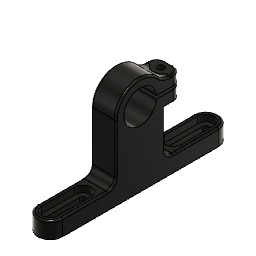
fixation (Autodesk Fusion 360 design; units mm, degrees)
Autodesk Fusion 360 part; units mm, degrees
sketch "Esquisse1" plane through (0, 0, 0) normal (1, 0, 0) x (0, 0, -1)
  circle A0 centre (0, 0) radius 10 construction
  circle A1 centre (0, 0) radius 15 construction
  line L0 (15, -35) -> (15, 0) construction
  line L1 (-15, -35) -> (-15, 0) construction
  line L2 (4, 1) -> (25, 1) construction
  line L3 (4, -1) -> (25, -1) construction
  line L4 (25, -1) -> (25, -7) construction
  line L5 (25, -7) -> (13.2665, -7) construction
  line L6 (25, 1) -> (25, 7) construction
  line L7 (25, 7) -> (13.2665, 7) construction
  line L8 (-15, -35) -> (-55, -35) construction
  line L9 (-55, -35) -> (-55, -45) construction
  line L10 (15, -35) -> (55, -35) construction
  line L11 (55, -35) -> (55, -45) construction
  line L12 (55, -45) -> (-55, -45) construction
  line L13 (55, -45) -> (-55, -45)
  line L14 (-55, -45) -> (-55, -35)
  line L15 (-55, -35) -> (-15, -35)
  line L16 (-15, -35) -> (-15, 0)
  line L17 (13.2665, 7) -> (25, 7)
  line L18 (25, 7) -> (25, 1)
  line L19 (25, 1) -> (9.9499, 1)
  line L20 (9.9499, -1) -> (25, -1)
  line L21 (25, -1) -> (25, -7)
  line L22 (25, -7) -> (15, -7)
  line L23 (15, -7) -> (15, -35)
  line L24 (15, -35) -> (55, -35)
  line L25 (55, -35) -> (55, -45)
  arc A2 (13.2665, 7) -> (-15, 0) centre (0, 0) ccw
  arc A3 (9.9499, 1) -> (9.9499, -1) centre (0, 0) ccw
  dimension "d58" = 20
  dimension "d59" = 30
  dimension "d60" = 10
  dimension "d61" = 10
  dimension "d62" = 45
  dimension "d63" = 10
  dimension "d64" = 10
  constraint coincident A0.centre A1.centre
  constraint coincident A1 L0.end
  constraint tangent A1 L0
  constraint vertical L0
  constraint coincident A1 L1.end
  constraint tangent A1 L1
  constraint parallel L0 L1
  constraint perpendicular L0 L2
  constraint horizontal L3
  constraint perpendicular L3 L4
  constraint coincident A1 L5.end
  constraint perpendicular L0 L5
  constraint perpendicular L2 L6
  constraint coincident A1 L7.end
  constraint perpendicular L6 L7
  constraint perpendicular L1 L8
  constraint perpendicular L8 L9
  constraint perpendicular L0 L10
  constraint perpendicular L10 L11
  constraint parallel L12 L13
  constraint coincident A0 L19.end
  constraint coincident L2 L19.end
  constraint coincident A0 L20.start
  constraint coincident L3 L20.start
  constraint coincident L5 L22.end
  constraint coincident L0 L22.end
  constraint parallel L11 L25
  measures "d58" diameter of A0
  measures "d59" diameter of A1
  measures "d60" distance of L0 L2.end
  measures "d61" distance of L0 L3.end
  measures "d62" distance of A0.centre L12
  measures "d63" distance of L10 L12
  measures "d64" distance of L8 L12
extrude "Extrusion8" add sketch "Esquisse1" along normal blind 15
fillet "Congé9" radius 7.5 4 edges at (15, -40, -55) (0, -40, -55) (15, -40, 55) (0, -40, 55)
fillet "Congé10" radius 5 2 edges at (7.5, -35, -15) (7.5, -35, 15)
sketch "Esquisse8" plane through (0, -35, 0) normal (0, 1, 0) x (-1, 0, 0)
  line L0 (-15, 20) -> (0, 20)
  line L1 (0, 20) -> (0, 47.5)
  arc A0 (0, 47.5) -> (-15, 47.5) centre (-7.5, 47.5) ccw
  line L2 (-15, 47.5) -> (-15, 20)
  line L3 (0, 47.5) -> (-15, 47.5) construction
  line L4 (-7.5, 55) -> (-7.5, 20) construction
  line L5 (0, 27.5) -> (-15, 27.5) construction
  line L6 (-2.5, 47.5) -> (-2.5, 27.5)
  line L7 (-5.5, 47.5) -> (-5.5, 27.5)
  arc A1 (-5.5, 47.5) -> (-7.5, 49.5) centre (-7.5, 47.5) ccw
  arc A2 (-2.5, 47.5) -> (-7.5, 52.5) centre (-7.5, 47.5) ccw
  arc A3 (-7.5, 25.5) -> (-5.5, 27.5) centre (-7.5, 27.5) ccw
  arc A4 (-7.5, 22.5) -> (-2.5, 27.5) centre (-7.5, 27.5) ccw
  arc A5 (-12.5, 27.5) -> (-7.5, 22.5) centre (-7.5, 27.5) ccw
  arc A6 (-9.5, 27.5) -> (-7.5, 25.5) centre (-7.5, 27.5) ccw
  line L8 (-9.5, 47.5) -> (-9.5, 27.5)
  line L9 (-12.5, 47.5) -> (-12.5, 27.5)
  arc A7 (-7.5, 52.5) -> (-12.5, 47.5) centre (-7.5, 47.5) ccw
  arc A8 (-7.5, 49.5) -> (-9.5, 47.5) centre (-7.5, 47.5) ccw
  line L10 (10, 0) -> (-30, 0)
  line L11 (-12.5, -47.5) -> (-12.5, -27.5)
  line L12 (-2.5, -47.5) -> (-2.5, -27.5)
  arc A9 (-7.5, -49.5) -> (-5.5, -47.5) centre (-7.5, -47.5) ccw
  arc A10 (-7.5, -52.5) -> (-2.5, -47.5) centre (-7.5, -47.5) ccw
  line L13 (-5.5, -47.5) -> (-5.5, -27.5)
  line L14 (0, -27.5) -> (-15, -27.5) construction
  arc A11 (-2.5, -27.5) -> (-7.5, -22.5) centre (-7.5, -27.5) ccw
  arc A12 (-5.5, -27.5) -> (-7.5, -25.5) centre (-7.5, -27.5) ccw
  arc A13 (-9.5, -47.5) -> (-7.5, -49.5) centre (-7.5, -47.5) ccw
  arc A14 (-12.5, -47.5) -> (-7.5, -52.5) centre (-7.5, -47.5) ccw
  line L15 (0, -47.5) -> (-15, -47.5) construction
  arc A15 (-7.5, -22.5) -> (-12.5, -27.5) centre (-7.5, -27.5) ccw
  line L16 (-9.5, -47.5) -> (-9.5, -27.5)
  arc A16 (-7.5, -25.5) -> (-9.5, -27.5) centre (-7.5, -27.5) ccw
  point P0 (-15, -47.5)
  point P1 (-7.5, -47.5)
  point P2 (0, -47.5)
  dimension "d71" = 20
  dimension "d72" = 5
  dimension "d73" = 2
  constraint coincident L1.end A0.start
  constraint coincident A0.end L2.start
  constraint midpoint A0 L4.start
  constraint midpoint L0 L4.end
  constraint coincident L1 L5.start
  constraint coincident L2 L5.end
  constraint perpendicular L2 L5
  constraint coincident L3 L6.start
  constraint coincident L5 L6.end
  constraint perpendicular L5 L6
  constraint coincident L3 L7.start
  constraint coincident L5 L7.end
  constraint perpendicular L5 L7
  constraint coincident A0.centre A1.centre
  constraint midpoint L5 A3.centre
  constraint coincident A3.centre A4.centre
  constraint symmetric L4 L6.start L9.start
  constraint symmetric L4 L6.end A5.start
  constraint symmetric L4 L7.start L8.start
  constraint symmetric L4 L7.end A6.start
  constraint symmetric L4 A1.end A8.start
  constraint symmetric L4 A1 A8
  constraint symmetric L4 A2.end A7.start
  constraint symmetric L4 A2 A7
  constraint symmetric L4 A3.start A6.end
  constraint symmetric L4 A3 A6
  constraint symmetric L4 A4.start A5.end
  constraint symmetric L4 A4 A5
  constraint horizontal L10
  constraint symmetric L1.end L10 P2
  constraint symmetric A0.end L10 P0
  constraint symmetric A0.centre L10 P1
  constraint symmetric L5.start L10 L14.start
  constraint symmetric L5.end L10 L14.end
  constraint symmetric L6.start L10 L12.start
  constraint symmetric L6.end L10 L12.end
  constraint symmetric L7.start L10 A9.end
  constraint symmetric L7.end L10 L13.end
  constraint symmetric A1.end L10 A9.start
  constraint symmetric A1 L10 A9
  constraint symmetric A2.end L10 A10.start
  constraint symmetric A2 L10 A10
  constraint symmetric A3.start L10 A12.end
  constraint symmetric A3 L10 A12
  constraint symmetric A4.start L10 A11.end
  constraint symmetric A4 L10 A11
  constraint symmetric A5.start L10 L11.end
  constraint symmetric A5 L10 A15
  constraint symmetric A6.start L10 L16.end
  constraint symmetric A6 L10 A16
  constraint symmetric L8.start L10 A13.start
  constraint symmetric L9.start L10 L11.start
  constraint symmetric A7 L10 A14
  constraint symmetric A8 L10 A13
  measures "d71" distance of L3 L5
  measures "d72" distance of L4 L6
  measures "d73" distance of L4 L7
extrude "Extrusion9" cut sketch "Esquisse8" against normal blind 20 contours L7 A1 A3 A6 L8 A8 | A9 L13 A12 A13 L16 A16
extrude "Extrusion10" cut sketch "Esquisse8" against normal blind 4 contours L6 A2 A4 A5 L9 A7 | L11 L12 A10 A11 A14 A15
sketch "Esquisse9" plane through (0, -7, 0) normal (0, -1, 0) x (1, 0, 0)
  line L0 (0, -15) -> (0, -25)
  line L1 (0, -25) -> (15, -25)
  line L2 (15, -25) -> (15, -15)
  line L3 (15, -15) -> (0, -15)
  line L4 (15, -25) -> (0, -15) construction
  line L5 (15, -15) -> (0, -25) construction
  circle A0 centre (7.5, -20) radius 2
  dimension "d78" = 4
  constraint coincident L1.end L2.start
  constraint coincident L0.start L3.end
  constraint coincident L2.end L3.start
  constraint coincident L0.end L1.start
  constraint midpoint L4 A0.centre
  measures "d78" diameter of A0
extrude "Extrusion11" cut sketch "Esquisse9" against normal blind 35 contours A0
fillet "Congé11" radius 10 1 edges at (7.5, 7, -13.2665)
ref_plane "Plan de construction2" through (7.5, 12, -19.1332) normal (0, 1, 0) x (0, 0, 1)
sketch "Esquisse10" plane through (7.5, 12, -21.6652) normal (0, 1, 0) x (1, 0, 0)
  arc A0 (1.101, -3.3348) -> (-1.101, -3.3348) centre (0, -1.6652) ccw
  circle A1 centre (0, -1.6652) radius 5
  dimension "d84" = 10
  constraint concentric A0 A1
  measures "d84" diameter of A1
extrude "Extrusion12" cut sketch "Esquisse10" against normal up to surface (5 mm away)
fillet "Congé12" radius 5 4 edges at (15, -4, -25) (15, 4, -25) (0, 4, -25) (0, -4, -25)
fillet "Congé13" radius 1 23 edges at (0, -15, 15) (0, -33.5355, 16.4645) (0, -35, 33.75) (7.5, -35, 55) (15, -35, 33.75) (15, -33.5355, 16.4645) (15, -15, 15) (15, 13.9638, 5.4785) (15, 7.8348, -14.3303) (15, 7, -19.1652) (13.5355, 7, -23.5355) (7.5, 7, -25) (1.4645, 7, -23.5355) (0, 7, -19.1652) (0, 7.8348, -14.3303) (0, 13.9638, 5.4785) (0, -18.5, -15) (0, -33.5355, -16.4645) (0, -35, -33.75) (7.5, -35, -55) (15, -35, -33.75) (15, -33.5355, -16.4645) (15, -18.5, -15)
